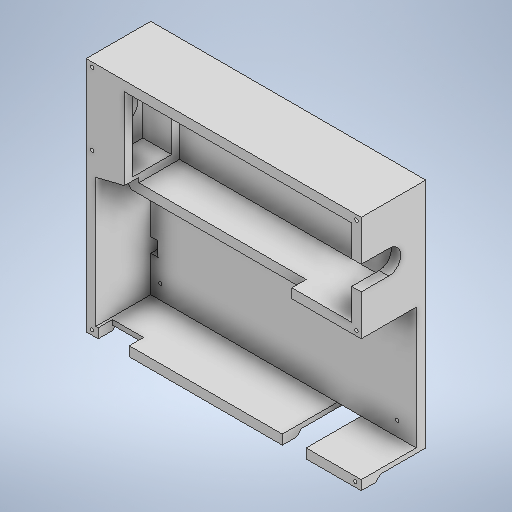
# Autodesk Inventor part: Honigschleuder_Steuerung_Netzteil
Saved by Autodesk Inventor 2025 (Build 290162010, 162A)
## iProperties
Created: 2025-12-06
Part Number: Honigschleuder_Steuerung_Netzteil
Material: Generisch
Document SubType Name: Modeling
Designer: max-h
Density: 1 g/cm^3
Appearance: Vorgabe
Author: max-h
Autodesk Inventor part; units mm, degrees
ref_plane "YZ Plane" through (0, 0, 0) normal (1, 0, 0) x (0, 1, 0)
ref_plane "XZ Plane" through (0, 0, 0) normal (0, 1, 0) x (-1, 0, 0)
ref_plane "XY Plane" through (0, 0, 0) normal (0, 0, 1) x (1, 0, 0)
sketch "Skizze1" plane through (0, 0, 0) normal (0, 0, 1) x (1, 0, 0)
  line L0 (0, 0) -> (115, 0)
  line L1 (115, 0) -> (115, -97)
  line L2 (115, -97) -> (0, -97)
  line L3 (0, -97) -> (0, 0)
  dimension "d0" = 115
  dimension "d1" = 97
  constraints: 8 end point, 2 parallel, 1 coincident, 1 horizontal, 1 perpendicular
  measures "d0" distance of L0.start L0.end
  measures "d1" distance of L2.end L0.start
extrude "Extrusion1" add sketch "Skizze1" along normal blind 4
sketch "Skizze2" plane through (0, 0, 4) normal (0, 0, 1) x (1, 0, 0)
  line L0 (0, -97) -> (115, -97) projected
  line L1 (115, -97) -> (115, 0) projected
  line L2 (115, 0) -> (0, 0) projected
  line L3 (0, 0) -> (0, -97) projected
  line L4 (4, -44) -> (4, -95)
  line L5 (4, -95) -> (115, -95)
  line L6 (115, -97) -> (115, 0) projected
  line L7 (4, -44) -> (115, -44)
  line L8 (4, -40) -> (16, -40) construction
  line L9 (4, -40) -> (4, -36.6) construction
  line L10 (4, -4) -> (16, -4) construction
  line L11 (4, -7.4) -> (16, -7.4)
  line L12 (16, -7.4) -> (16, -4)
  line L13 (4, -36.6) -> (16, -36.6)
  line L14 (16, -36.6) -> (16, -40)
  line L15 (4, -36.6) -> (4, -7.4)
  line L16 (16, -40) -> (111, -40)
  line L17 (4, -7.4) -> (4, -4) construction
  line L18 (16, -4) -> (111, -4)
  line L19 (111, -4) -> (111, -40)
  point P0 (109.25, 0)
  point P1 (109.25, -40)
  dimension "d4" = 4
  dimension "d5" = 2
  dimension "d6" = 51
  dimension "d7" = 4
  dimension "d8" = 36
  dimension "d9" = 4
  dimension "d10" = 29.2
  dimension "d11" = 12
  dimension "d30" = 4
  constraints: 30 end point, 12 perpendicular, 4 horizontal, 4 point on line, 4 vertical, 2 equal length
  measures "d4" distance between parallel lines of L3 L4
  measures "d5" distance between parallel lines of L0 L5
  measures "d6" distance of L4.start L4.end
  measures "d7" distance between parallel lines of L7 L8
  measures "d8" distance of L8.start L10.start
  measures "d9" distance between parallel lines of L3 L9
  measures "d10" distance between parallel lines of L13 L11
  measures "d11" distance of L11.start L11.end
  measures "d30" distance between parallel lines of L6 L19
extrude "Extrusion2" add sketch "Skizze2" along normal blind 23 contours L3 L2 L1 L7 L4 L5 L0
sketch "Skizze4" plane through (0, 0, 4) normal (0, 0, 1) x (1, 0, 0)
  line L0 (4, -36.6) -> (16, -36.6) projected
  line L1 (4, -36.6) -> (16, -36.6)
  line L2 (16, -36.6) -> (16, -7.4)
  line L3 (16, -7.4) -> (4, -7.4)
  line L4 (4, -7.4) -> (4, -36.6)
  point P0 (0, 0)
  point P1 (16, -7.4)
  constraints: 8 end point, 2 parallel, 1 coincident, 1 horizontal, 1 perpendicular
extrude "Extrusion4" add sketch "Skizze4" along normal blind 3.3
sketch "Skizze5" plane through (4, -36.6, 27) normal (1, 0, 0) x (0, 0, -1)
  line L0 (0, 0) -> (0, 29.2) projected
  line L1 (0, 29.2) -> (3.3, 29.2)
  line L2 (3.3, 29.2) -> (3.3, 0)
  line L3 (3.3, 0) -> (0, 0)
  line L4 (0, 0) -> (0, 29.2)
  line L5 (19.7, 0) -> (0, 0) projected
  line L6 (19.7, 0) -> (19.7, 29.2) projected
  circle A0 centre (11.5, 14.6) radius 6.1
  line L7 (7.2229, 14.6) -> (16.7001, 14.6)
  line L8 (11.5, 24.1317) -> (11.5, 8.2548) construction
  point P0 (27, 36.6)
  dimension "d20" = 16.4
  dimension "d21" = 29.2
  dimension "d22" = 12.2
  constraints: 12 end point, 3 point on line, 2 horizontal, 2 parallel, 1 centre point, 1 perpendicular, 1 vertical, 1 other
  measures "d20" distance between parallel lines of L6 L2
  measures "d21" diameter of L5 L7
  measures "d22" diameter of A0
extrude "Extrusion5" cut sketch "Skizze5" against normal through all contours A0
extrude "Extrusion6" add sketch "Skizze5" along normal up to surface (12 mm away) contours L0 L1 L2 L3
sketch "Skizze6" plane through (0, 0, 27) normal (0, 0, 1) x (1, 0, 0)
  line L0 (4, -44) -> (115, -44) projected
  line L1 (111, -40) -> (16, -40) projected
  line L2 (86, -44) -> (16, -44)
  line L3 (16, -44) -> (16, -40)
  line L4 (16, -40) -> (86, -40)
  line L5 (86, -40) -> (86, -44)
  line L6 (4, -44) -> (4, -95) projected
  line L7 (0, -97) -> (115, -97) projected
  line L8 (14, -97) -> (7, -97)
  line L9 (115, -95) -> (4, -95) projected
  line L10 (92, -95) -> (82, -95)
  line L11 (82, -95) -> (82, -97)
  line L12 (82, -97) -> (92, -97)
  line L13 (92, -97) -> (92, -95)
  line L14 (115, -97) -> (115, -95) projected
  line L15 (5, -95) -> (18, -95)
  line L16 (18, -95) -> (18, -97)
  line L17 (18, -97) -> (5, -97)
  line L18 (5, -97) -> (5, -95)
  line L19 (0, 0) -> (0, -97) projected
  point P0 (109.25, -40)
  point P1 (86, -42)
  point P2 (86, -40)
  point P3 (82, -95)
  point P4 (5, -96)
  point P5 (18, -96)
  point P6 (5, -97)
  point P7 (18, -97)
  dimension "d27" = 70
  dimension "d41" = 10
  dimension "d42" = 23
  dimension "d65" = 13
  dimension "d66" = 5
  constraints: 26 end point, 6 parallel, 6 point on line, 3 horizontal, 3 midpoint, 3 perpendicular
  measures "d27" distance from line of point (86, -42) L3
  measures "d41" distance between parallel lines of L13 L11
  measures "d42" distance between parallel lines of L14 L13
  measures "d65" distance of point (5, -96) point (18, -96)
  measures "d66" distance between parallel lines of L19 L18
extrude "Extrusion7" cut sketch "Skizze6" against normal blind 6 contours L3 L1 L5 L0
sketch "Skizze7" plane through (115, -97, 0) normal (1, 0, 0) x (0, 0, -1)
  arc A0 (-15.5, 80) -> (-15.5, 70) centre (-15.5, 75) ccw construction
  circle A1 centre (-15.5, 75) radius 6.1 construction
  line L0 (-15.5, 80) -> (-27, 80)
  line L1 (-27, 53) -> (-27, 97) projected
  line L2 (-15.5, 70) -> (-27, 70)
  arc A2 (-15.5, 70) -> (-15.5, 80) centre (-15.5, 75) ccw
  point P0 (0, 97)
  dimension "d31" = 10
  constraints: 4 end point, 4 point on circle, 2 centre point, 2 horizontal, 2 point on line, 2 tangent, 1 coincident
  measures "d31" diameter of A0
extrude "Extrusion8" cut sketch "Skizze7" against normal blind 4
sketch "Skizze8" plane through (0, 0, 0) normal (0, 0, -1) x (-1, 0, 0)
  line L0 (0, -97) -> (-115, -97) projected
  line L1 (0, 0) -> (0, -97) projected
  line L2 (-115, 0) -> (0, 0) projected
  line L3 (-115, -97) -> (-115, 0) projected
  line L4 (-8, -8) -> (-8, -89) construction
  line L5 (-8, -89) -> (-107, -89) construction
  line L6 (-107, -89) -> (-107, -8) construction
  line L7 (-107, -8) -> (-8, -8) construction
  circle A0 centre (-107, -89) radius 0.7
  circle A1 centre (-8, -89) radius 0.7
  circle A2 centre (-103, -8) radius 0.7
  circle A3 centre (-12, -8) radius 0.7
  line L8 (-107, -8) -> (-8, -89) construction
  line L9 (-107, -89) -> (-8, -8) construction
  circle A4 centre (-57.5, -48.5) radius 0.7
  dimension "d34" = 8
  dimension "d35" = 1.4
  dimension "d36" = 4
  dimension "d37" = 4
  constraints: 12 end point, 5 centre point, 4 equal radius, 2 coincident, 2 point on line, 1 midpoint, 3 other
  measures "d34" distance between parallel lines of L2 L7
  measures "d35" diameter of A2
  measures "d36" distance from line of L6 A2.centre
  measures "d37" distance from line of L4 A3.centre
extrude "Extrusion9" cut sketch "Skizze8" against normal blind 4 contours A0 | A1 | A2 | A3 | A4
extrude "Extrusion10" cut sketch "Skizze6" against normal blind 6 contours L9 L16 L7 L18
sketch "Skizze9" plane through (0, 0, 27) normal (0, 0, 1) x (1, 0, 0)
  line L0 (4, -95) -> (4, -44) projected
  line L1 (4, -44) -> (16, -44) projected
  line L2 (16, -44) -> (16, -4) projected
  line L3 (16, -4) -> (111, -4) projected
  line L4 (111, -4) -> (111, -17) projected
  line L5 (111, -40) -> (86, -40) projected
  line L6 (86, -40) -> (86, -44) projected
  line L7 (86, -44) -> (115, -44) projected
  line L8 (115, -44) -> (115, -27) projected
  line L9 (115, 0) -> (0, 0) projected
  line L10 (0, 0) -> (0, -97) projected
  line L11 (0, -97) -> (5, -97) projected
  line L12 (2.5, -2) -> (113, -2) construction
  line L13 (113, -2) -> (113, -97.1903) construction
  line L14 (113, -97.1903) -> (2.5, -97.1903) construction
  line L15 (2.5, -97.1903) -> (2.5, -2) construction
  circle A0 centre (2.5, -2) radius 0.7
  circle A1 centre (113, -2) radius 0.7
  circle A2 centre (113, -42) radius 0.7
  line L16 (113, -42) -> (2.5, -42) construction
  line L17 (4, -44) -> (16, -44) construction
  circle A3 centre (2.5, -32) radius 0.7
  line L18 (115, -27) -> (111, -27) projected
  line L19 (111, -27) -> (111, -40) projected
  line L20 (111, -17) -> (115, -17) projected
  line L21 (115, -17) -> (115, 0) projected
  line L22 (115, -97) -> (115, -95) projected
  line L23 (115, -95) -> (18, -95) projected
  line L24 (5, -97) -> (5, -95) projected
  line L25 (5, -95) -> (4, -95) projected
  line L26 (18, -95) -> (18, -97) projected
  line L27 (18, -97) -> (115, -97) projected
  dimension "d45" = 2
  dimension "d46" = 2.5
  dimension "d47" = 2
  dimension "d48" = 1.4
  dimension "d49" = 2
  dimension "d59" = 30
  constraints: 10 end point, 4 centre point, 3 parallel, 3 point on line, 2 coincident, 2 equal radius, 1 horizontal, 1 perpendicular
  measures "d45" distance between parallel lines of L9 L12
  measures "d46" distance between parallel lines of L10 L15
  measures "d47" distance between parallel lines of L8 L13
  measures "d48" diameter of A0
  measures "d49" distance between parallel lines of L7 L16
  measures "d59" distance of L12.start A3.centre
extrude "Extrusion11" cut sketch "Skizze9" against normal blind 4 contours A0 | A1 | A2 | A3
extrude "Extrusion12" cut sketch "Skizze6" against normal through all contours L9 L13 L7 L11
sketch "Skizze12" plane through (0, -97, 0) normal (0, -1, 0) x (1, 0, 0)
  line L0 (115, 4) -> (115, 27) projected
  line L1 (115, 27) -> (92, 27)
  line L2 (92, 27) -> (92, 21)
  line L3 (92, 21) -> (115, 21)
  line L4 (115, 21) -> (115, 27)
  line L5 (82, 0) -> (82, 27) projected
  line L6 (18, 27) -> (18, 21) projected
  line L7 (82, 27) -> (18, 27)
  line L8 (18, 27) -> (18, 21)
  line L9 (18, 21) -> (82, 21)
  line L10 (82, 21) -> (82, 27)
  line L11 (5, 21) -> (5, 27) projected
  line L12 (0, 0) -> (0, 27) projected
  line L13 (5, 21) -> (0, 21)
  line L14 (0, 21) -> (0, 27)
  line L15 (0, 27) -> (5, 27)
  line L16 (5, 27) -> (5, 21)
  point P0 (5, 27)
  point P1 (0, 21)
  dimension "d67" = 6
  constraints: 24 end point, 7 parallel, 3 horizontal, 3 perpendicular, 3 point on line, 1 coincident
  measures "d67" distance between parallel lines of L1 L3
extrude "Extrusion15" add sketch "Skizze12" along normal blind 2
sketch "Skizze10" plane through (0, 0, 27) normal (0, 0, 1) x (1, 0, 0)
  line L0 (16, -44) -> (16, -4) projected
  line L1 (4, -44) -> (16, -44) projected
  line L2 (4, -95) -> (4, -44) projected
  line L3 (4, -44) -> (4, -41)
  line L4 (4, -41) -> (16, -38)
  point P0 (0, 0)
  dimension "d56" = 6
  dimension "d77" = 3
  constraints: 4 end point, 1 point on line, 1 vertical
  measures "d56" distance of L0.start L4.end
  measures "d77" distance of L1.start L3.end
extrude "Extrusion13" cut sketch "Skizze10" against normal blind 6
sketch "Skizze11" plane through (0, 0, 4) normal (0, 0, 1) x (1, 0, 0)
  circle A0 centre (12, -52) radius 1.2
  line L0 (4, -44) -> (4, -95) projected
  line L1 (115, -44) -> (4, -44) projected
  point P0 (0, 0)
  dimension "d60" = 8
  dimension "d61" = 8
  dimension "d62" = 2.4
  constraints: 1 centre point
  measures "d60" distance from line of L0 A0.centre
  measures "d61" distance from line of L1 A0.centre
  measures "d62" diameter of A0
extrude "Extrusion14" cut sketch "Skizze11" against normal blind 4
sketch "Skizze13" plane through (0, 0, 27) normal (0, 0, 1) x (1, 0, 0)
  line L0 (5, -97) -> (0, -97) projected
  circle A0 centre (2.5, -97) radius 0.7
  circle A1 centre (2.5, -32) radius 0.7 projected
  line L1 (0, 0) -> (0, -99) projected
  line L2 (115, -97) -> (92, -97) projected
  circle A2 centre (112.5, -97) radius 0.7
  line L3 (115, -95) -> (115, -99) projected
  dimension "d70" = 2.5
  dimension "d71" = 2.5
  constraints: 2 centre point, 2 equal radius, 1 midpoint, 1 point on line
  measures "d70" distance from line of L1 A0.centre
  measures "d71" distance from line of L3 A2.centre
extrude "Extrusion16" cut sketch "Skizze13" against normal blind 5 contours A0 L0 | L0 A0 | A2 L2 | L2 A2
chamfer "Fasen1" distance 2 angle 45 3 edges at (2.5, -97, 21) (50, -97, 21) (103.5, -97, 21)
sketch "Skizze14" plane through (0, 0, 4) normal (0, 0, 1) x (1, 0, 0)
  line L0 (115, -44) -> (4, -44) projected
  line L1 (4, -74) -> (7, -74)
  line L2 (7, -74) -> (7, -80)
  line L3 (7, -80) -> (4, -80)
  line L4 (4, -80) -> (4, -44)
  line L5 (4, -95) -> (82, -95) projected
  point P0 (0, 0)
  point P1 (7, -44)
  point P2 (4, -74)
  dimension "d78" = 6
  dimension "d79" = 3
  dimension "d82" = 15
  constraints: 8 end point, 2 parallel, 1 horizontal, 1 perpendicular
  measures "d78" distance of L1.end L2.end
  measures "d79" distance of L2.end L3.end
  measures "d82" distance between parallel lines of L5 L3
extrude "Extrusion17" cut sketch "Skizze14" against normal blind 10
sketch "Skizze16" plane through (0, 0, 21) normal (0, 0, 1) x (1, 0, 0)
  line L0 (86, -44) -> (4, -44) projected
  line L1 (4, -44) -> (4, -41) projected
  line L2 (4, -44) -> (4, -41)
  line L3 (4, -41) -> (9, -39.75)
  line L4 (4, -41) -> (16, -38) projected
  line L5 (9, -44.0784) -> (9, -39.75)
  point P0 (0, 0)
  point P1 (9, -41.9142)
  point P2 (9, -44)
  dimension "d83" = 5
  constraints: 6 end point, 1 collinear, 1 midpoint, 1 perpendicular, 1 point on line
  measures "d83" distance from line of point (9, -41.914) L1
extrude "Extrusion18" cut sketch "Skizze16" against normal up to surface (17 mm away)
chamfer "Fasen2" distance 4 angle 45 1 edges at (9, -44, 12.5)
